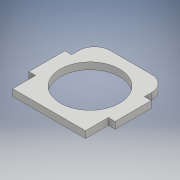
# Autodesk Inventor part: muñeca3
Saved by Autodesk Inventor 2018 (Build 220112000, 112)
## iProperties
Created: 2020-03-11
Part Number: muñeca3
Material: Genérico
Document SubType Name: Modeling
Designer: david
Density: 1 g/cm^3
Appearance: Valor por defecto
Author: david
Autodesk Inventor part; units mm, degrees
ref_plane "YZ Plane" through (0, 0, 0) normal (1, 0, 0) x (0, 1, 0)
ref_plane "XZ Plane" through (0, 0, 0) normal (0, 1, 0) x (-1, 0, 0)
ref_plane "XY Plane" through (0, 0, 0) normal (0, 0, 1) x (1, 0, 0)
sketch "Boceto1" plane through (0, 0, 0) normal (0, 0, 1) x (1, 0, 0)
  circle A0 centre (0, 0) radius 13.175
  line L0 (0, -18.175) -> (-16.175, -18.175)
  line L1 (-9.175, 18.175) -> (9.175, 18.175)
  line L2 (16.175, -18.175) -> (0, -18.175)
  line L3 (-19.175, 0) -> (-19.175, 8)
  line L4 (-19.175, 8) -> (-16.175, 8)
  line L5 (-19.175, 0) -> (-19.175, -8)
  line L6 (-19.175, -8) -> (-16.175, -8)
  line L7 (-16.175, -18.175) -> (-16.175, -8)
  line L8 (-16.175, 8) -> (-16.175, 11.175)
  line L9 (16.175, -8) -> (19.175, -8)
  line L10 (19.175, -8) -> (19.175, 8)
  line L11 (19.175, 8) -> (16.175, 8)
  line L12 (16.175, 11.175) -> (16.175, 8)
  line L13 (16.175, -8) -> (16.175, -18.175)
  arc A1 (-9.175, 18.175) -> (-16.175, 11.175) centre (-9.175, 11.175) ccw
  arc A2 (16.175, 11.175) -> (9.175, 18.175) centre (9.175, 11.175) ccw
  dimension "d12" = 7
  dimension "d15" = 32.35
  dimension "d16" = 29.35
  dimension "d17" = 8
  dimension "d18" = 10.175
  constraints: 28 end point, 14 perpendicular, 4 point on circle, 4 tangent, 3 centre point, 2 horizontal, 2 point on line, 1 equal radius
  measures "d12" radius of A1
  measures "d15" distance between parallel lines of L13 L7
  measures "d16" distance of L8.end L0.end
  measures "d17" distance of L3.start L5.end
  measures "d18" distance of L0.end L6.end
extrude "Extrusión1" add sketch "Boceto1" along normal blind 3
